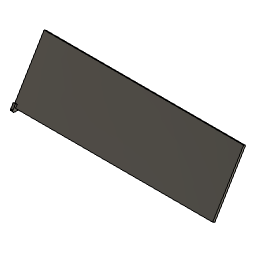
Desk Stand (Autodesk Fusion 360 design; units mm, degrees)
Autodesk Fusion 360 part; units mm, degrees
sketch "Sketch1" plane through (0, 0, 0) normal (0, 1, 0) x (1, 0, 0) in component "Board"
  line L0 (0, 0) -> (300, 0)
  line L1 (300, 0) -> (300, -90)
  line L2 (300, -90) -> (0, -90)
  line L3 (0, -90) -> (0, 0)
  dimension "d1" = 300
  dimension "d2" = 90
  constraint horizontal L0
  constraint vertical L1
  constraint horizontal L2
  constraint vertical L3
  constraint coincident L0.start L3.end
  measures "d1" distance of L0.start L0.end
  measures "d2" distance of L0.start L2.end
extrude "Extrude1" add sketch "Sketch1" against normal blind 3.4 makes body 1 in component "Board"
move_body "Move1" bodies 1 to x (1, 0, 0) y (0, 0.857167, -0.515038) z (0, 0.515038, 0.857167) at (0, 0, 0) in component "Board"
sketch "Sketch1 (2)" plane through (0, 0, 0) normal (1, 0, 0) x (0, 1, 0) in component "Stand"
  line L0 (46.3534, 77.1451) -> (0, 0)
  line L1 (43.4391, 78.8962) -> (-2.9144, 1.7511)
  line L2 (0, 0) -> (-2.9144, 1.7511)
  line L3 (0, 0) -> (-5.4859, 3.2962)
  line L4 (-5.4859, 3.2962) -> (-7.031, 0.7247)
  line L5 (-7.031, 0.7247) -> (-1.5451, -2.5715)
  line L6 (-1.5451, -2.5715) -> (0, 0)
  line L7 (-2.9144, 1.7511) -> (-5.4859, 3.2962)
  line L8 (-5.4859, 3.2962) -> (-2.9107, 7.5821)
  line L9 (-2.9107, 7.5821) -> (-0.3392, 6.037)
  line L10 (-0.3392, 6.037) -> (-2.9144, 1.7511)
  line L11 (36.1075, 60.093) -> (33.4549, 55.6783)
  line L12 (33.4549, 55.6783) -> (40.8022, 51.2635)
  line L13 (40.8022, 51.2635) -> (43.4549, 55.6783)
  line L14 (43.4549, 55.6783) -> (36.1075, 60.093)
  line L15 (-1.5451, -2.5715) -> (43.4549, -2.5715)
  line L16 (43.4549, -2.5715) -> (43.4549, 5.4285)
  line L17 (43.4549, 5.4285) -> (-1.5451, 5.4285)
  line L18 (-1.5451, 5.4285) -> (-1.5451, -2.5715)
  line L19 (43.4549, 55.6783) -> (33.4549, 55.6783)
  line L20 (33.4549, 55.6783) -> (33.4549, 5.4285)
  line L21 (33.4549, 5.4285) -> (43.4549, 5.4285)
  line L22 (43.4549, 5.4285) -> (43.4549, 55.6783)
  line L23 (3.2618, 5.4285) -> (-1.5451, -2.5715)
  line L24 (-1.5451, -2.5715) -> (-7.031, -2.5715)
  line L25 (-7.031, -2.5715) -> (-7.031, 0.7247)
  dimension "d5" = 3
  dimension "d6" = 5
  dimension "d7" = 3
  dimension "d8" = 45
  dimension "d9" = 8
  dimension "d10" = 10
  constraint perpendicular L3 L4
  constraint parallel L3 L5
  constraint parallel L4 L6
  constraint perpendicular L1 L3
  constraint coincident L0.end L2.start
  constraint perpendicular L7 L8
  constraint parallel L7 L9
  constraint parallel L8 L10
  constraint perpendicular L4 L7
  constraint coincident L1.end L2.end
  constraint perpendicular L11 L12
  constraint parallel L11 L13
  constraint parallel L12 L14
  constraint coincident L0 L11.end
  constraint parallel L0 L11
  constraint horizontal L15
  constraint vertical L16
  constraint horizontal L17
  constraint vertical L18
  constraint horizontal L19
  constraint vertical L20
  constraint horizontal L21
  constraint vertical L22
  constraint coincident L17 L20.end
  constraint collinear L16 L22
  constraint coincident L12 L11.end
  constraint coincident L11.end L12.start
  constraint coincident L17 L23.start
  constraint coincident L0 L23.start
  constraint perpendicular L18 L24
  constraint perpendicular L24 L25
  measures "d5" distance of L3.end L4.end
  measures "d6" distance of L3.end L8.end
  measures "d7" distance of L8.end L9.end
  measures "d8" distance of L5.end L15.end
  measures "d9" distance of L15.end L16.end
  measures "d10" distance of L13.end L11.end
extrude "Extrude1'" add sketch "Sketch1 (2)" along normal blind 3.4 separate body contours L0 L11 L14 L19 | L12 L13 L19 | L12 L13 L17 L20 L21 L22 | L0 L6 L15 L16 L17 L21 L23 | L2 L3 L6 L18 L23 | L1 L3 L7 L8 L9 L10 L17 L18 | L1 L10 L17 L18 | L2 L3 L4 L5 L7 L18 | L5 L24 L25 makes body 2 in component "Stand"
fillet "Fillet1" radius 10 1 edges at (1.7, 33.4549, 5.4285) on bodies 2 in component "Stand"
fillet "Fillet2" radius 2.5 3 edges at (1.7, 43.4549, -2.5715) (1.7, 43.4549, 55.6783) (1.7, -7.031, -2.5715) on bodies 2 in component "Stand"
fillet "Fillet3" radius 2 1 edges at (1.7, -7.031, 0.7247) on bodies 2 in component "Stand"
component "Board" placed x (1, 0, 0) y (0, 1, 0) z (0, 0, 1) at (0, 0, 0)
component "Stand" placed x (1, 0, 0) y (0, 1, 0) z (0, 0, 1) at (0, 0, 0)
